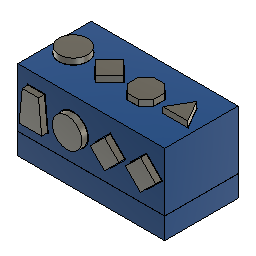
Version 2 (Autodesk Fusion 360 design; units mm, degrees)
Autodesk Fusion 360 part; units mm, degrees
note: some values were not read from the file. Chosen so that the rebuilt part matches the saved one: which face or edge a step refers to; which pieces of a blend or face edit are solid. Set by a fixed rule: which sketch regions a step uses.
sketch "Sketch1" plane through (0, 0, 0) normal (0, 0, 1) x (1, 0, 0)
  line L0 (0, 0) -> (200, 0)
  line L1 (200, 0) -> (200, 100)
  line L2 (200, 100) -> (0, 100)
  line L3 (0, 100) -> (0, 0)
  dimension "d1" = 200
  dimension "d2" = 100
  constraint horizontal L0
  constraint vertical L1
  constraint horizontal L2
  constraint vertical L3
  constraint coincident L0.start L3.end
  measures "d1" distance of L0.start L0.end
  measures "d2" distance of L0.start L2.end
extrude "Extrude1" add sketch "Sketch1" along normal blind 30 makes body 1
sketch "Sketch2" plane through (0, 0, 30) normal (0, 0, 1) x (-1, 0, 0)
  line L0 (0, -100) -> (0, 0)
  line L1 (0, 0) -> (-200, 0)
  line L2 (-200, 0) -> (-200, -100)
  line L3 (-200, -100) -> (0, -100)
  line L4 (0, -100) -> (-10, -100)
  line L5 (-10, -100) -> (-10, -90)
  line L6 (-10, -90) -> (0, -90)
  line L7 (0, -90) -> (0, -100)
  line L8 (-200, 0) -> (-190, 0)
  line L9 (-190, 0) -> (-190, -10)
  line L10 (-190, -10) -> (-200, -10)
  line L11 (-200, -10) -> (-200, 0)
  line L12 (-10, -90) -> (-190, -90)
  line L13 (-190, -90) -> (-190, -10)
  line L14 (-190, -10) -> (-10, -10)
  line L15 (-10, -10) -> (-10, -90)
  dimension "d5" = 10
  dimension "d6" = 10
  dimension "d7" = 10
  dimension "d8" = 10
  constraint horizontal L4
  constraint vertical L5
  constraint horizontal L6
  constraint vertical L7
  constraint coincident L0.start L3.end
  constraint horizontal L8
  constraint vertical L9
  constraint horizontal L10
  constraint vertical L11
  constraint coincident L1.end L2.start
  constraint horizontal L12
  constraint vertical L13
  constraint horizontal L14
  constraint vertical L15
  measures "d5" distance of L0.start L4.end
  measures "d6" distance of L0.start L6.end
  measures "d7" distance of L1.end L8.end
  measures "d8" distance of L1.end L10.end
extrude "Extrude2" add sketch "Sketch2" along normal blind 15 contours L12 L13 L14 L15 bodies 1
sketch "Sketch3" plane through (0, 0, 45) normal (0, 0, 1) x (-1, 0, 0)
  line L0 (-10, -10) -> (-190, -10)
  line L1 (-190, -10) -> (-190, -90)
  line L2 (-190, -90) -> (-10, -90)
  line L3 (-10, -90) -> (-10, -10)
  line L4 (-10, -10) -> (-16, -10)
  line L5 (-16, -10) -> (-16, -16)
  line L6 (-16, -16) -> (-10, -16)
  line L7 (-10, -16) -> (-10, -10)
  line L8 (-190, -90) -> (-184, -90)
  line L9 (-184, -90) -> (-184, -84)
  line L10 (-184, -84) -> (-190, -84)
  line L11 (-190, -84) -> (-190, -90)
  line L12 (-184, -84) -> (-16, -84)
  line L13 (-16, -84) -> (-16, -16)
  line L14 (-16, -16) -> (-184, -16)
  line L15 (-184, -16) -> (-184, -84)
  dimension "d11" = 6
  dimension "d12" = 6
  dimension "d13" = 6
  dimension "d14" = 6
  constraint horizontal L4
  constraint vertical L5
  constraint horizontal L6
  constraint vertical L7
  constraint coincident L0.start L3.end
  constraint horizontal L8
  constraint vertical L9
  constraint horizontal L10
  constraint vertical L11
  constraint coincident L1.end L2.start
  constraint horizontal L12
  constraint vertical L13
  constraint horizontal L14
  constraint vertical L15
  measures "d11" distance of L0.start L4.end
  measures "d12" distance of L0.start L6.end
  measures "d13" distance of L1.end L8.end
  measures "d14" distance of L1.end L10.end
extrude "Extrude3" cut sketch "Sketch3" against normal blind 35 contours L12 L13 L14 L15 bodies 1
ref_plane "WorkPlane1" through (100, 50, 45) normal (0, 0, 1) x (1, 0, 0)
sketch "Sketch4" plane through (0, 0, 45) normal (0, 0, 1) x (1, 0, 0)
  line L0 (0, 0) -> (200, 0)
  line L1 (200, 0) -> (200, 100)
  line L2 (200, 100) -> (0, 100)
  line L3 (0, 100) -> (0, 0)
  constraint horizontal L0
  constraint vertical L1
  constraint horizontal L2
  constraint vertical L3
  constraint coincident L0.start L3.end
extrude "Extrude4" add sketch "Sketch4" along normal blind 100 separate body makes body 2
extrude "Extrude5" add 1 faces at (70, 3.3333, 30) along direction (0, 0, 1) blind 16 separate body on bodies 1 makes body 3
combine "Combine1" operation add target body 2 tool bodies 3
extrude "Extrude6" cut 1 faces at (128, 61.3333, 10) along direction (0, 0, 1) blind 130 on bodies 1 bodies 2
move_face "OffsetFaces1" offset -0.1 4 faces at (70, 90, 40) (190, 63.3333, 35) (130, 10, 40) (10, 36.6667, 35) on bodies 2
extrude "Extrude7" cut 1 faces at (69.9667, 96.7, 30) along direction (0, 0, 1) blind 0.2 on bodies 2 bodies 2
extrude "Extrude8" cut 1 faces at (128, 11.9333, 45) along direction (0, 0, 1) blind 0.2 on bodies 2 bodies 2
extrude "Extrude9" cut 1 faces at (72, 16, 76.8) along direction (0, -1, 0) blind 6.1 on bodies 2 bodies 2
extrude "Extrude10" cut 1 faces at (128, 84, 76.8) along direction (0, 1, 0) blind 6.1 on bodies 2 bodies 2
extrude "Extrude11" cut 1 faces at (16, 36.6333, 108.4) along direction (-1, 0, 0) blind 6.1 on bodies 2 bodies 2
extrude "Extrude12" cut 1 faces at (184, 63.3667, 76.8) along direction (1, 0, 0) blind 6.1 on bodies 2 bodies 2
extrude "Extrude13" add 1 faces at (69.9667, 36.6333, 140) along direction (0, 0, -1) blind 5 on bodies 2 bodies 2
sketch "Sketch5" plane through (0, 100, 0) normal (0, 1, 0) x (-1, 0, 0)
  line L0 (-200, 0) -> (0, 0)
  line L1 (0, 0) -> (0, 30)
  line L2 (0, 30) -> (-200, 30)
  line L3 (-200, 30) -> (-200, 0)
  line L4 (-200, 30) -> (-192, 30)
  line L5 (-192, 30) -> (-192, 22)
  line L6 (-192, 22) -> (-200, 22)
  line L7 (-200, 22) -> (-200, 30)
  line L8 (0, 0) -> (-8, 0)
  line L9 (-8, 0) -> (-8, 8)
  line L10 (-8, 8) -> (0, 8)
  line L11 (0, 8) -> (0, 0)
  line L12 (-192, 22) -> (-8, 22)
  line L13 (-8, 22) -> (-8, 8)
  line L14 (-8, 8) -> (-192, 8)
  line L15 (-192, 8) -> (-192, 22)
  dimension "d39" = 8
  dimension "d40" = 8
  dimension "d41" = 8
  dimension "d42" = 8
  constraint horizontal L4
  constraint vertical L5
  constraint horizontal L6
  constraint vertical L7
  constraint coincident L2.end L3.start
  constraint horizontal L8
  constraint vertical L9
  constraint horizontal L10
  constraint vertical L11
  constraint coincident L0.end L1.start
  constraint horizontal L12
  constraint vertical L13
  constraint horizontal L14
  constraint vertical L15
  measures "d39" distance of L2.end L4.end
  measures "d40" distance of L2.end L6.end
  measures "d41" distance of L0.end L8.end
  measures "d42" distance of L0.end L10.end
extrude "Extrude14" cut sketch "Sketch5" against normal blind 6 contours L12 L13 L14 L15 bodies 1
extrude "Extrude15" add 1 faces at (69.3333, 94, 12.6667) along direction (0, 1, 0) blind 2 on bodies 1 bodies 1
fillet "Fillet1" radius 6 1 faces at (69.3333, 96, 12.6667) on bodies 1
delete_face "DeleteFace1" 1 faces at (71.219, 96, 14.5523) on bodies 1
delete_face "DeleteFace2" 1 faces at (129.2276, 96.2885, 18.1812) on bodies 1
delete_face "DeleteFace3" 1 faces at (8.7658, 98.5247, 12.1235) on bodies 1
fillet "Fillet2" radius 5 1 faces at (128, 61.3333, 10) on bodies 1
fillet "Fillet3" radius 3 1 faces at (69.9667, 36.6333, 135) on bodies 2
chamfer "Chamfer1" distance 1 angle 45 1 faces at (66.6667, 66.6667, 145) on bodies 2
fillet "Fillet4" radius 4 4 edges at (190, 50, 45) (100, 10, 45) (100, 90, 45) (10, 50, 45) on bodies 1
chamfer "Chamfer2" distance 1 angle 45 1 faces at (66.6667, 66.6667, 0) on bodies 1
sketch "Sketch6" plane through (0, 0, 145) normal (0, 0, 1) x (-1, 0, 0)
  line L0 (-199, -1) -> (-199, -99)
  line L1 (-199, -99) -> (-1, -99)
  line L2 (-1, -99) -> (-1, -1)
  line L3 (-1, -1) -> (-199, -1)
  line L4 (-174.5, -70) -> (-157.1795, -40)
  line L5 (-157.1795, -40) -> (-191.8205, -40)
  line L6 (-191.8205, -40) -> (-174.5, -70)
  line L7 (-55.0001, -49.9341) -> (-75.0659, -30.0001)
  line L8 (-75.0659, -30.0001) -> (-94.9999, -50.0659)
  line L9 (-94.9999, -50.0659) -> (-74.9341, -69.9999)
  line L10 (-74.9341, -69.9999) -> (-55.0001, -49.9341)
  circle A0 centre (-25.5, -50) radius 20
  line L11 (-50, -50) -> (-45.5, -50)
  line L12 (-5.5, -50) -> (-1, -50)
  line L13 (-5.5, -50) -> (-1, -50)
  line L14 (-55.0656, -50) -> (-45.5, -50)
  line L15 (-50, -50) -> (-55.0656, -50)
  line L16 (-94.9344, -50) -> (-100, -50)
  line L17 (-100, -50) -> (-105, -50)
  line L18 (-145, -50) -> (-150, -50)
  line L19 (-105, -50) -> (-94.9344, -50)
  line L20 (-150, -50) -> (-162.953, -50)
  line L21 (-186.047, -50) -> (-199, -50)
  line L22 (-199, -50) -> (-186.047, -50)
  line L23 (-162.953, -50) -> (-145, -50)
  point P0 (-174.5, -50)
  point P1 (-125, -50)
  point P2 (-75, -50)
  dimension "d57" = 20
  dimension "d58" = 20
  dimension "d59" = 20
  dimension "d60" = 40
  constraint midpoint L0 L21.end
  constraint midpoint L2 L12.end
  constraint coincident L11.start L22
  constraint perpendicular L2 L15
  constraint coincident L18.end L22
  constraint coincident L17.end L22
  constraint coincident A0 L11.end
  constraint coincident A0 L12.start
  constraint collinear L11 L12
  constraint coincident A0.centre L11
  constraint collinear L13 L22
  constraint coincident L16.end L22
  constraint coincident L8 L16.start
  constraint coincident L10 L14.start
  constraint collinear L14 L22
  constraint collinear L15 L16
  constraint coincident P2 L15
  constraint collinear L17 L18
  constraint coincident P1 L17
  constraint collinear L19 L22
  constraint coincident L4 L20.end
  constraint coincident L6 L21.start
  constraint collinear L20 L21
  constraint coincident P0 L20
  constraint collinear L22 L23
  measures "d57" distance of L4.start P0
  measures "d58" distance of L17.end P1
  measures "d59" distance of L7.start P2
  measures "d60" diameter of A0
extrude "Extrude16" cut sketch "Sketch6" against normal blind 30 contours L4 L5 L6 | L7 L8 L9 L10 | A0 bodies 2
sketch "Sketch7" plane through (0, 0, 145) normal (0, 0, 1) x (-1, 0, 0)
  line L0 (-157.1795, -40) -> (-174.5, -70)
  line L1 (-174.5, -70) -> (-191.8205, -40)
  line L2 (-191.8205, -40) -> (-157.1795, -40)
  line L3 (-75.0659, -30.0001) -> (-55.0001, -49.9341)
  line L4 (-55.0001, -49.9341) -> (-74.9341, -69.9999)
  line L5 (-74.9341, -69.9999) -> (-94.9999, -50.0659)
  line L6 (-94.9999, -50.0659) -> (-75.0659, -30.0001)
  circle A0 centre (-25.5, -50) radius 20
  line L7 (-199, -1) -> (-199, -99)
  line L8 (-199, -99) -> (-1, -99)
  line L9 (-1, -99) -> (-1, -1)
  line L10 (-1, -1) -> (-199, -1)
  line L11 (-25.5, -50) -> (-174.5, -50)
  line L12 (-199, -50) -> (-124.5, -50)
  line L13 (-124.5, -50) -> (-124.5, -30) construction
  line L14 (-124.5, -50) -> (-104.5, -50) construction
  line L15 (-124.5, -50) -> (-106.0224, -42.3463) construction
  line L16 (-124.5, -50) -> (-104.5, -50) construction
  line L17 (-106.0224, -42.3463) -> (-116.8463, -31.5224)
  line L18 (-116.8463, -31.5224) -> (-132.1537, -31.5224)
  line L19 (-132.1537, -31.5224) -> (-142.9776, -42.3463)
  line L20 (-142.9776, -42.3463) -> (-142.9776, -57.6537)
  line L21 (-142.9776, -57.6537) -> (-132.1537, -68.4776)
  line L22 (-132.1537, -68.4776) -> (-116.8463, -68.4776)
  line L23 (-116.8463, -68.4776) -> (-106.0224, -57.6537)
  line L24 (-106.0224, -57.6537) -> (-106.0224, -42.3463)
  point P0 (-124.5, -50)
  dimension "d63" = 74.5
  dimension "d64" = 20
  dimension "d65" = 20
  dimension "d66" = 22.5
  dimension "d67" = 20
  constraint coincident A0.centre L11.start
  constraint parallel L2 L11
  constraint midpoint L7 L12.start
  constraint perpendicular L9 L12
  constraint vertical L13
  constraint horizontal L14
  constraint horizontal L16
  constraint coincident L15.end L17.start
  constraint coincident P0 L12.end
  measures "d63" distance of L12.start P0
  measures "d64" distance of P0 L13.end
  measures "d65" distance of P0 L14.end
  measures "d66" angle of L15 L16
  measures "d67" distance of P0 L15.end
extrude "Extrude17" cut sketch "Sketch7" against normal blind 5 contours L11 L12 L20 L21 L22 L23 L24 | L11 L12 L17 L18 L19 L20 L24 bodies 2
extrude "Extrude18" cut 1 faces at (127.0512, 43.8408, 140) along direction (0, 0, -1) blind 10 on bodies 2 bodies 2
extrude "Extrude19" cut 1 faces at (9.9, 45.8281, 58.4667) along direction (-1, 0, 0) blind 5 on bodies 2 bodies 2
extrude "Extrude20" cut 1 faces at (7.7184, 38.2235, 115) along direction (0, 0, 1) blind 20 on bodies 2 bodies 2
delete_face "DeleteFace4" 2 faces at (12.3792, 20.0516, 134.9545) (8.2333, 19.0948, 132) on bodies 2
delete_face "DeleteFace5" 2 faces at (12.5182, 79.9395, 134.9756) (8.2333, 71.7104, 132) on bodies 2
delete_face "DeleteFace6" 1 faces at (128.1311, 10.2169, 133.3419) on bodies 2
delete_face "DeleteFace7" 1 faces at (190.0966, 29.9667, 132.1427) on bodies 2
delete_face "DeleteFace8" 1 faces at (187.5509, 60.8922, 134.9659) on bodies 2
extrude "Extrude21" cut 1 faces at (190.1, 47.66, 58.4667) along direction (1, 0, 0) blind 5 on bodies 2 bodies 2
extrude "Extrude22" cut 1 faces at (192.3402, 41.9867, 115) along direction (0, 0, 1) blind 20 on bodies 2 bodies 2
delete_face "DeleteFace9" 2 faces at (66.6333, 87.2427, 134.9966) (193.4333, 90.0966, 132.1427) on bodies 2
extrude "Extrude23" cut 1 faces at (131.7, 9.9, 100.0667) along direction (0, -1, 0) blind 5 on bodies 2 bodies 2
extrude "Extrude24" cut 1 faces at (131.7, 90.1, 65.1333) along direction (0, 1, 0) blind 5 on bodies 2 bodies 2
delete_face "DeleteFace10" 1 faces at (71.3333, 86.5076, 44.9677) on bodies 1
delete_face "DeleteFace11" 1 faces at (128.6667, 13.4924, 44.9677) on bodies 1
delete_face "DeleteFace12" 1 faces at (13.8097, 63.3333, 44.9955) on bodies 1
delete_face "DeleteFace13" 1 faces at (188.8949, 63.3333, 43.7603) on bodies 1
move_face "OffsetFaces2" offset 5 4 faces at (10, 36.6667, 35) (130, 10, 40) (190, 63.3333, 35) (70, 90, 40) on bodies 1
move_face "OffsetFaces3" offset -5 4 faces at (72, 16, 35) (184, 38.6667, 25) (128, 84, 35) (16, 61.3333, 35) on bodies 1
move_face "OffsetFaces4" offset 35 1 faces at (91.6886, 13.2667, 135) on bodies 2
delete_face "DeleteFace14" 1 faces at (133, 99.6667, 144.3333) on bodies 2
delete_face "DeleteFace15" 2 faces at (133, 0.3333, 144.3333) (199.6667, 33.6667, 144.3333) on bodies 2
delete_face "DeleteFace16" 1 faces at (0.6667, 66.6667, 144.6667) on bodies 2
extrude "Extrude25" cut 1 faces at (91.6886, 10, 145) along direction (0, 0, -1) blind 35 on bodies 2 bodies 2
sketch "Sketch8" plane through (0, 0, 110) normal (0, 0, 1) x (-1, 0, 0)
  circle A0 centre (-25.5, -50) radius 20
  line L0 (-75.0659, -30.0001) -> (-55.0001, -49.9341)
  line L1 (-55.0001, -49.9341) -> (-74.9341, -69.9999)
  line L2 (-74.9341, -69.9999) -> (-94.9999, -50.0659)
  line L3 (-94.9999, -50.0659) -> (-75.0659, -30.0001)
  line L4 (-157.1795, -40) -> (-174.5, -70)
  line L5 (-174.5, -70) -> (-191.8205, -40)
  line L6 (-191.8205, -40) -> (-157.1795, -40)
  line L7 (-116.8463, -31.5224) -> (-106.0224, -42.3463)
  line L8 (-106.0224, -42.3463) -> (-106.0224, -57.6537)
  line L9 (-106.0224, -57.6537) -> (-116.8463, -68.4776)
  line L10 (-116.8463, -68.4776) -> (-132.1537, -68.4776)
  line L11 (-132.1537, -68.4776) -> (-142.9776, -57.6537)
  line L12 (-142.9776, -57.6537) -> (-142.9776, -42.3463)
  line L13 (-142.9776, -42.3463) -> (-132.1537, -31.5224)
  line L14 (-132.1537, -31.5224) -> (-116.8463, -31.5224)
  line L15 (0, -100) -> (0, 0)
  line L16 (0, 0) -> (-200, 0)
  line L17 (-200, 0) -> (-200, -100)
  line L18 (-200, -100) -> (0, -100)
  circle A1 centre (-25.5, -50) radius 19.5
  dimension "d89" = 39
  constraint concentric A0 A1
  measures "d89" diameter of A1
extrude "Extrude26" add sketch "Sketch8" along normal blind 10 separate body contours A1 makes body 4
sketch "Sketch9" plane through (0, 0, 110) normal (0, 0, 1) x (-1, 0, 0)
  circle A0 centre (-25.5, -50) radius 20
  line L0 (-75.0659, -30.0001) -> (-55.0001, -49.9341)
  line L1 (-55.0001, -49.9341) -> (-74.9341, -69.9999)
  line L2 (-74.9341, -69.9999) -> (-94.9999, -50.0659)
  line L3 (-94.9999, -50.0659) -> (-75.0659, -30.0001)
  line L4 (-157.1795, -40) -> (-174.5, -70)
  line L5 (-174.5, -70) -> (-191.8205, -40)
  line L6 (-191.8205, -40) -> (-157.1795, -40)
  line L7 (-116.8463, -31.5224) -> (-106.0224, -42.3463)
  line L8 (-106.0224, -42.3463) -> (-106.0224, -57.6537)
  line L9 (-106.0224, -57.6537) -> (-116.8463, -68.4776)
  line L10 (-116.8463, -68.4776) -> (-132.1537, -68.4776)
  line L11 (-132.1537, -68.4776) -> (-142.9776, -57.6537)
  line L12 (-142.9776, -57.6537) -> (-142.9776, -42.3463)
  line L13 (-142.9776, -42.3463) -> (-132.1537, -31.5224)
  line L14 (-132.1537, -31.5224) -> (-116.8463, -31.5224)
  line L15 (0, -100) -> (0, 0)
  line L16 (0, 0) -> (-200, 0)
  line L17 (-200, 0) -> (-200, -100)
  line L18 (-200, -100) -> (0, -100)
  line L19 (-94.5, -50.0286) -> (-74.9714, -69.5)
  line L20 (-74.9714, -69.5) -> (-55.5, -49.9714)
  line L21 (-55.5, -49.9714) -> (-75.0286, -30.5)
  line L22 (-75.0286, -30.5) -> (-94.5, -50.0286)
  point P0 (-75, -50)
  dimension "d92" = 19.5
  measures "d92" distance of L19.start P0
extrude "Extrude27" add sketch "Sketch9" along normal blind 10 separate body contours L19 L20 L21 L22 makes body 5
sketch "Sketch10" plane through (0, 0, 110) normal (0, 0, 1) x (-1, 0, 0)
  circle A0 centre (-25.5, -50) radius 20
  line L0 (-75.0659, -30.0001) -> (-55.0001, -49.9341)
  line L1 (-55.0001, -49.9341) -> (-74.9341, -69.9999)
  line L2 (-74.9341, -69.9999) -> (-94.9999, -50.0659)
  line L3 (-94.9999, -50.0659) -> (-75.0659, -30.0001)
  line L4 (-157.1795, -40) -> (-174.5, -70)
  line L5 (-174.5, -70) -> (-191.8205, -40)
  line L6 (-191.8205, -40) -> (-157.1795, -40)
  line L7 (-116.8463, -31.5224) -> (-106.0224, -42.3463)
  line L8 (-106.0224, -42.3463) -> (-106.0224, -57.6537)
  line L9 (-106.0224, -57.6537) -> (-116.8463, -68.4776)
  line L10 (-116.8463, -68.4776) -> (-132.1537, -68.4776)
  line L11 (-132.1537, -68.4776) -> (-142.9776, -57.6537)
  line L12 (-142.9776, -57.6537) -> (-142.9776, -42.3463)
  line L13 (-142.9776, -42.3463) -> (-132.1537, -31.5224)
  line L14 (-132.1537, -31.5224) -> (-116.8463, -31.5224)
  line L15 (0, -100) -> (0, 0)
  line L16 (0, 0) -> (-200, 0)
  line L17 (-200, 0) -> (-200, -100)
  line L18 (-200, -100) -> (0, -100)
  circle A1 centre (0, 100) radius 20
  line L19 (-13.0656, 86.9344) -> (-14.1421, 85.8579)
  line L20 (0, 100) -> (20, 100) construction
  line L21 (-18.4776, 92.3463) -> (-7.6537, 81.5224)
  line L22 (-7.6537, 81.5224) -> (7.6537, 81.5224)
  line L23 (7.6537, 81.5224) -> (18.4776, 92.3463)
  line L24 (18.4776, 92.3463) -> (18.4776, 107.6537)
  line L25 (18.4776, 107.6537) -> (7.6537, 118.4776)
  line L26 (7.6537, 118.4776) -> (-7.6537, 118.4776)
  line L27 (-7.6537, 118.4776) -> (-18.4776, 107.6537)
  line L28 (-18.4776, 107.6537) -> (-18.4776, 92.3463)
  point P0 (0, 100)
  dimension "d95" = 40
  dimension "d96" = 135
  constraint horizontal L20
  constraint coincident P0 A1.centre
  constraint coincident L21 L19.start
  measures "d95" diameter of A1
  measures "d96" angle of L19 L20
extrude "Extrude28" add sketch "Sketch10" along normal blind 10 separate body contours L21 L22 L23 L24 L25 L26 L27 L28 makes body 6
move_body "Move1" bodies 6 to x (1, 0, 0) y (0, 1, 0) z (0, 0, 1) at (124.5, 150, 0)
move_face "OffsetFaces5" offset -0.25 9 faces at (106.0224, 52.5512, 116.6667) (113.2384, 64.8696, 116.6667) (127.0512, 68.4776, 113.3333) (135.7616, 64.8696, 113.3333) (141.1736, 59.4577, 113.3333) (142.9776, 47.4488, 116.6667) (135.7616, 35.1304, 113.3333) (121.9488, 31.5224, 116.6667) (109.6304, 38.7384, 113.3333) on bodies 6
extrude "Extrude29" cut 3 faces at (120.2037, 45.7037, 120) (75.0095, 43.5, 120) (20.8078, 46.5477, 120) along direction (0, 0, -1) blind 2 on bodies 4 5 6 bodies 4 5 6
sketch "Sketch11" plane through (0, 0, 110) normal (0, 0, 1) x (-1, 0, 0)
  circle A0 centre (-25.5, -50) radius 20
  line L0 (-75.0659, -30.0001) -> (-55.0001, -49.9341)
  line L1 (-55.0001, -49.9341) -> (-74.9341, -69.9999)
  line L2 (-74.9341, -69.9999) -> (-94.9999, -50.0659)
  line L3 (-94.9999, -50.0659) -> (-75.0659, -30.0001)
  line L4 (-157.1795, -40) -> (-174.5, -70)
  line L5 (-174.5, -70) -> (-191.8205, -40)
  line L6 (-191.8205, -40) -> (-157.1795, -40)
  line L7 (-116.8463, -31.5224) -> (-106.0224, -42.3463)
  line L8 (-106.0224, -42.3463) -> (-106.0224, -57.6537)
  line L9 (-106.0224, -57.6537) -> (-116.8463, -68.4776)
  line L10 (-116.8463, -68.4776) -> (-132.1537, -68.4776)
  line L11 (-132.1537, -68.4776) -> (-142.9776, -57.6537)
  line L12 (-142.9776, -57.6537) -> (-142.9776, -42.3463)
  line L13 (-142.9776, -42.3463) -> (-132.1537, -31.5224)
  line L14 (-132.1537, -31.5224) -> (-116.8463, -31.5224)
  line L15 (0, -100) -> (0, 0)
  line L16 (0, 0) -> (-200, 0)
  line L17 (-200, 0) -> (-200, -100)
  line L18 (-200, -100) -> (0, -100)
  line L19 (-0.0017, 30.5) -> (16.8884, 59.7485)
  line L20 (16.8884, 59.7485) -> (-16.8866, 59.7515)
  line L21 (-16.8866, 59.7515) -> (-0.0017, 30.5)
  point P0 (0, 50)
  dimension "d103" = 19.5
  measures "d103" distance of L19.start P0
extrude "Extrude30" add sketch "Sketch11" along normal blind 8 separate body contours L19 L20 L21 makes body 7
move_body "Move2" bodies 7 to x (1, 0, 0) y (0, 1, 0) z (0, 0, 1) at (174.5009, 99.75, 0)
sketch "Sketch12" plane through (0, 100, 0) normal (0, 1, 0) x (-1, 0, 0)
  line L0 (0, 110) -> (-200, 110)
  line L1 (-200, 110) -> (-200, 30.2)
  line L2 (-200, 30.2) -> (0, 30.2)
  line L3 (0, 30.2) -> (0, 110)
  line L4 (-200, 70.1) -> (0, 70.1) construction
  line L5 (-200, 70.1) -> (-150, 70.1) construction
  line L6 (-150, 70.1) -> (-100, 70.1) construction
  line L7 (-100, 70.1) -> (-50, 70.1) construction
  line L8 (-50, 70.1) -> (0, 70.1) construction
  line L9 (-160, 95.1) -> (-190, 95.1) construction
  line L10 (-190, 95.1) -> (-190, 45.1) construction
  line L11 (-190, 45.1) -> (-160, 45.1) construction
  line L12 (-160, 45.1) -> (-160, 95.1) construction
  line L13 (-160, 95.1) -> (-190, 45.1) construction
  line L14 (-190, 95.1) -> (-160, 45.1) construction
  line L15 (-160, 45.1) -> (-190, 45.1)
  line L16 (-190, 45.1) -> (-190, 95.1)
  line L17 (-190, 95.1) -> (-160, 95.1)
  line L18 (-160, 95.1) -> (-160, 45.1)
  line L19 (-160, 45.1) -> (-190, 95.1) construction
  line L20 (-190, 45.1) -> (-160, 95.1) construction
  line L21 (-105, 52.6) -> (-145, 52.6)
  line L22 (-145, 52.6) -> (-145, 87.6)
  line L23 (-145, 87.6) -> (-105, 87.6)
  line L24 (-105, 87.6) -> (-105, 52.6)
  line L25 (-105, 52.6) -> (-145, 87.6) construction
  line L26 (-145, 52.6) -> (-105, 87.6) construction
  line L27 (-75, 70.1) -> (-75, 80.1)
  line L28 (-75, 100.1) -> (-92.3205, 70.1)
  line L29 (-92.3205, 70.1) -> (-57.6795, 70.1)
  line L30 (-57.6795, 70.1) -> (-75, 100.1)
  line L31 (-92.3205, 70.1) -> (-57.6795, 70.1)
  line L32 (-57.6795, 70.1) -> (-57.6795, 52.1)
  line L33 (-57.6795, 52.1) -> (-92.3205, 52.1)
  line L34 (-92.3205, 52.1) -> (-92.3205, 70.1)
  line L35 (-3.3494, 57.6) -> (-25, 95.1)
  line L36 (-25, 95.1) -> (-46.6506, 57.6)
  line L37 (-46.6506, 57.6) -> (-3.3494, 57.6)
  line L38 (-161, 46.1) -> (-189, 46.1)
  line L39 (-189, 46.1) -> (-189, 94.1)
  line L40 (-189, 94.1) -> (-161, 94.1)
  line L41 (-161, 94.1) -> (-161, 46.1)
  line L42 (-106, 86.6) -> (-106, 53.6)
  line L43 (-106, 53.6) -> (-144, 53.6)
  line L44 (-144, 53.6) -> (-144, 86.6)
  line L45 (-144, 86.6) -> (-106, 86.6)
  line L46 (-58.6795, 69.8321) -> (-75, 98.1)
  line L47 (-75, 98.1) -> (-91.3205, 69.8321)
  line L48 (-91.3205, 53.1) -> (-91.3205, 69.8321)
  line L49 (-58.6795, 53.1) -> (-91.3205, 53.1)
  line L50 (-58.6795, 69.8321) -> (-58.6795, 53.1)
  line L51 (-5.0814, 58.6) -> (-25, 93.1)
  line L52 (-25, 93.1) -> (-44.9186, 58.6)
  line L53 (-44.9186, 58.6) -> (-5.0814, 58.6)
  point P0 (-175, 70.1)
  point P1 (-175, 70.1)
  point P2 (-125, 70.1)
  point P3 (-75, 80.1)
  point P4 (-25, 70.1)
  dimension "d106" = 30
  dimension "d107" = 50
  dimension "d108" = 40
  dimension "d109" = 35
  dimension "d110" = 10
  dimension "d111" = 20
  dimension "d112" = 18
  dimension "d113" = 12.5
  dimension "d116" = 1
  dimension "d117" = 1
  dimension "d118" = 1
  dimension "d119" = -1
  constraint midpoint L1 L4.start
  constraint midpoint L3 L4.end
  constraint coincident L4 L5.end
  constraint perpendicular L1 L5
  constraint midpoint L4 L6.end
  constraint perpendicular L1 L6
  constraint coincident L4 L7.end
  constraint horizontal L9
  constraint perpendicular L9 L10
  constraint parallel L9 L11
  constraint parallel L10 L12
  constraint coincident L13 P1
  constraint coincident L14 P1
  constraint midpoint L5 P1
  constraint horizontal L15
  constraint perpendicular L15 L16
  constraint parallel L15 L17
  constraint parallel L16 L18
  constraint coincident L19 P1
  constraint coincident L20 P1
  constraint coincident P1 P0
  constraint horizontal L21
  constraint perpendicular L21 L22
  constraint parallel L21 L23
  constraint parallel L22 L24
  constraint coincident L25 P2
  constraint coincident L26 P2
  constraint midpoint L6 P2
  constraint midpoint L7 L27.start
  constraint perpendicular L7 L27
  constraint coincident P3 L27.end
  constraint horizontal L31
  constraint vertical L32
  constraint horizontal L33
  constraint vertical L34
  constraint midpoint L8 P4
  measures "d106" distance of L10.end L11.end
  measures "d107" distance of L9.end L10.end
  measures "d108" distance of L22.end L23.end
  measures "d109" distance of L21.end L22.end
  measures "d110" distance of L27.start P3
  measures "d111" distance of L28.start P3
  measures "d112" distance of L28.end L33.end
  measures "d113" distance of P4 L37
extrude "Extrude31" cut sketch "Sketch12" against normal blind 20 contours L15 L16 L17 L18 | L21 L22 L23 L24 | L28 L29 L30 L31 L46 L47 | L29 L31 L32 L33 L34 L46 L47 L48 L49 L50 | L29 L31 L46 L47 | L29 L31 L46 L47 L48 L49 L50 | L35 L36 L37 | L38 L39 L40 L41 | L42 L43 L44 L45 | L51 L52 L53 bodies 2
extrude "Extrude32" add sketch "Sketch12" along normal blind 8 separate body contours L29 L31 L46 L47 | L29 L31 L46 L47 L48 L49 L50 | L38 L39 L40 L41 | L42 L43 L44 L45 | L51 L52 L53 makes body 8 at (75, 100, 79.2547) makes body 9 at (131.3333, 100, 75.6) makes body 10 at (25, 100, 70.1) makes body 11 at (170.3333, 100, 62.1)
extrude "Extrude33" cut 1 faces at (134.1038, 86.2259, 100) along direction (0, 0, 1) blind 5 on bodies 2 bodies 2
extrude "Extrude34" cut 1 faces at (75.0577, 85.0333, 101.6667) along direction (-1, 0, 0) blind 3 on bodies 2 bodies 2
sketch "Sketch13" plane through (0, 0, 0) normal (0, -1, 0) x (1, 0, 0)
  line L0 (200, 110) -> (0, 110)
  line L1 (0, 110) -> (0, 30.2)
  line L2 (0, 30.2) -> (200, 30.2)
  line L3 (200, 30.2) -> (200, 110)
  line L4 (50, 70.1) -> (100, 70.1) construction
  line L5 (100, 70.1) -> (150, 70.1) construction
  line L6 (150, 70.1) -> (200, 70.1) construction
  line L7 (41.5, 47.6) -> (8.5, 47.6)
  line L8 (13, 92.6) -> (37, 92.6)
  line L9 (41.5, 47.6) -> (8.5, 92.6) construction
  line L10 (8.5, 47.6) -> (37.54, 87.2) construction
  line L11 (25, 92.6) -> (13, 92.6)
  line L12 (13, 92.6) -> (8.5, 47.6)
  line L13 (25, 92.6) -> (37, 92.6)
  line L14 (37, 92.6) -> (41.5, 47.6)
  line L15 (13.905, 91.6) -> (36.095, 91.6)
  line L16 (36.095, 91.6) -> (40.395, 48.6)
  line L17 (40.395, 48.6) -> (9.605, 48.6)
  line L18 (13.905, 91.6) -> (9.605, 48.6)
  line L19 (0, 70.1) -> (10.75, 70.1) construction
  line L20 (39.25, 70.1) -> (50, 70.1) construction
  line L21 (0, 70.1) -> (10.75, 70.1)
  line L22 (39.25, 70.1) -> (200, 70.1)
  dimension "d127" = 45
  dimension "d128" = 12
  dimension "d129" = 1
  constraint midpoint L1 L19.start
  constraint midpoint L3 L6.end
  constraint coincident L4.start L21
  constraint perpendicular L1 L4
  constraint coincident L5.end L21
  constraint horizontal L7
  constraint parallel L7 L8
  constraint parallel L8 L11
  constraint parallel L8 L13
  constraint coincident L14 L10.end
  constraint coincident L8 L11.start
  constraint collinear L19 L20
  constraint collinear L21 L22
  constraint coincident L4.end L21
  constraint coincident L12 L19.end
  constraint coincident L14 L20.start
  measures "d127" distance of L7.end L9.end
  measures "d128" distance of L11.start L8.end
extrude "Extrude35" cut sketch "Sketch13" against normal blind 5 contours L7 L8 L11 L12 L13 L14 | L15 L16 L17 L18 bodies 2
extrude "Extrude36" add sketch "Sketch13" along normal blind 8 separate body contours L15 L16 L17 L18 makes body 12
sketch "Sketch14" plane through (0, 0, 0) normal (0, -1, 0) x (1, 0, 0)
  line L0 (8.5, 47.6) -> (13, 92.6)
  line L1 (13, 92.6) -> (37, 92.6)
  line L2 (37, 92.6) -> (41.5, 47.6)
  line L3 (41.5, 47.6) -> (8.5, 47.6)
  line L4 (200, 110) -> (0, 110)
  line L5 (0, 110) -> (0, 30.2)
  line L6 (0, 30.2) -> (200, 30.2)
  line L7 (200, 30.2) -> (200, 110)
  line L8 (0, 70.1) -> (200, 70.1)
  line L9 (50, 70.1) -> (100, 70.1)
  circle A0 centre (75, 70.1) radius 21
  circle A1 centre (75, 70.1) radius 20
  dimension "d134" = 42
  dimension "d137" = -1
  constraint midpoint L5 L8.start
  constraint midpoint L7 L8.end
  constraint horizontal L9
  constraint coincident L8 L9.start
  constraint midpoint L9 A0.centre
  measures "d134" diameter of A0
extrude "Extrude37" cut sketch "Sketch14" against normal blind 5 contours L8 L9 A0 A1 | L8 L9 A0 A1 | L8 L9 A1 | L8 L9 A1 bodies 2
extrude "Extrude38" add sketch "Sketch14" along normal blind 8 separate body contours L8 L9 A1 | L8 L9 A1 makes body 13
sketch "Sketch15" plane through (0, 0, 0) normal (0, -1, 0) x (1, 0, 0)
  circle A0 centre (75, 70.1) radius 21
  line L0 (8.5, 47.6) -> (13, 92.6)
  line L1 (13, 92.6) -> (37, 92.6)
  line L2 (37, 92.6) -> (41.5, 47.6)
  line L3 (41.5, 47.6) -> (8.5, 47.6)
  line L4 (200, 110) -> (0, 110)
  line L5 (0, 110) -> (0, 30.2)
  line L6 (0, 30.2) -> (200, 30.2)
  line L7 (200, 30.2) -> (200, 110)
  line L8 (200, 70.1) -> (100, 70.1)
  line L9 (100, 70.1) -> (150, 70.1)
  line L10 (146.9967, 70.1) -> (125.9967, 91.1)
  line L11 (125.9967, 91.1) -> (104.9967, 70.1)
  line L12 (104.9967, 70.1) -> (125.9967, 49.1)
  line L13 (125.9967, 49.1) -> (146.9967, 70.1)
  line L14 (150, 70.1) -> (200, 70.1)
  line L15 (196.9985, 69.8448) -> (175.2552, 92.0985)
  line L16 (175.2552, 92.0985) -> (153.0015, 70.3552)
  line L17 (153.0015, 70.3552) -> (174.7448, 48.1015)
  line L18 (174.7448, 48.1015) -> (196.9985, 69.8448)
  line L19 (106.4109, 70.1) -> (125.9967, 50.5142)
  line L20 (125.9967, 50.5142) -> (145.5825, 70.1)
  line L21 (145.5825, 70.1) -> (125.9967, 89.6858)
  line L22 (125.9967, 89.6858) -> (106.4109, 70.1)
  line L23 (154.4156, 70.3388) -> (174.7612, 49.5156)
  line L24 (174.7612, 49.5156) -> (195.5844, 69.8612)
  line L25 (195.5844, 69.8612) -> (175.2388, 90.6844)
  line L26 (175.2388, 90.6844) -> (154.4156, 70.3388)
  point P0 (125.9967, 70.1)
  point P1 (175, 70.1)
  dimension "d140" = 21
  dimension "d141" = 22
  dimension "d144" = -1
  dimension "d145" = -1
  constraint midpoint L7 L8.start
  constraint perpendicular L7 L8
  constraint midpoint L8 L9.end
  constraint coincident L9 P0
  constraint perpendicular L7 L14
  constraint midpoint L14 P1
  measures "d140" distance of L10.start P0
  measures "d141" distance of L15.start P1
extrude "Extrude39" cut sketch "Sketch15" against normal blind 5 contours L8 L9 L12 L13 L19 L20 | L8 L9 L10 L11 L21 L22 | L8 L9 L19 L20 | L8 L9 L21 L22 | L8 L14 L15 L17 L18 L23 L24 L25 | L8 L14 L15 L16 L17 L23 L25 L26 | L8 L14 L23 L24 L25 | L8 L14 L23 L25 L26 bodies 2
extrude "Extrude40" add sketch "Sketch15" along normal blind 8 separate body contours L8 L9 L19 L20 | L8 L9 L21 L22 | L8 L14 L23 L24 L25 | L8 L14 L23 L25 L26 makes body 14 at (125.9967, 0, 76.6286) makes body 15 at (168.1385, 0, 70.1796)
move_face "MoveFace1" by (3, 0, 0) 2 faces at (39.4338, 96.7333, 70.1) (11.0831, 98.3667, 70.9953) on bodies 2
move_body "Move3" bodies 10 to x (1, 0, 0) y (0, 1, 0) z (0, 0, 1) at (3, 0, 0)
